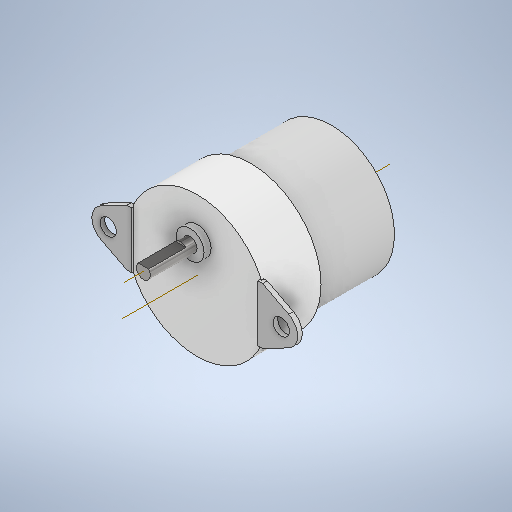
# Autodesk Inventor part: SPG27
Saved by Autodesk Inventor 2025.3 (Build 293356030, 356C)
## iProperties
Created: 2025-08-17
Part Number: SPG27
Material: 一般
Document SubType Name: Modeling
Designer: daisuke
Density: 1 g/cm^3
Appearance: 既定
Author: daisuke
Autodesk Inventor part; units mm, degrees
ref_plane "YZ Plane" through (0, 0, 0) normal (1, 0, 0) x (0, 1, 0)
sketch "スケッチ1" plane through (0, 0, 0) normal (0, 0, 1) x (1, 0, 0)
  circle A0 centre (0, 0) radius 15
  dimension "d0" = 30
  constraints: 1 centre point, 1 coincident
  measures "d0" diameter of A0
extrude "押し出し1" add sketch "スケッチ1" against normal blind 11.5
sketch "スケッチ2" plane through (0, 0, 0) normal (0, 0, 1) x (1, 0, 0)
  circle A0 centre (0, 6.5) radius 3
  point P0 (0, 0)
  dimension "d3" = 6
  dimension "d4" = 6.5
  constraints: 1 centre point, 1 vertical alignment
  measures "d3" diameter of A0
  measures "d4" distance of point (0, 0) A0.centre
extrude "押し出し2" add sketch "スケッチ2" along normal blind 1.5
sketch "スケッチ3" plane through (0, 6.5, 1.5) normal (0, 0, 1) x (1, 0, 0)
  circle A0 centre (0, 0) radius 3 projected
  circle A1 centre (0, 0) radius 1.5
  point P0 (0, -6.5)
  dimension "d7" = 3
  constraints: 1 centre point, 1 coincident
  measures "d7" diameter of A1
extrude "押し出し3" add sketch "スケッチ3" along normal blind 10 contours A1
sketch "スケッチ4" plane through (0, 0, -11.5) normal (0, 0, -1) x (-1, 0, 0)
  circle A0 centre (0, 0) radius 13.5
  dimension "d10" = 27
  constraints: 1 centre point, 1 coincident
  measures "d10" diameter of A0
extrude "押し出し4" add sketch "スケッチ4" along normal blind 17.2
sketch "スケッチ6" plane through (0, 6.5, 11.5) normal (0, 0, 1) x (1, 0, 0)
  circle A0 centre (0, 0) radius 1.5 projected
  line L0 (-1.118, 1) -> (1.118, 1)
  point P0 (0, -6.5)
  dimension "d21" = 1
  constraints: 2 end point, 2 point on circle, 1 horizontal
  measures "d21" distance from line of L0 A0.centre
extrude "押し出し6" cut sketch "スケッチ6" against normal blind 8 contours L0 A0 picked at (-0.0599, 1.1631)
ref_plane "作業平面1" through (0, 0, 0.5) normal (0, 0, 1) x (1, 0, 0)
sketch "スケッチ7" plane through (0, 0, 0.5) normal (0, 0, 1) x (1, 0, 0)
  line L0 (0, 21.4774) -> (0, -21.4774) construction
  line L1 (-14.5, 6) -> (-13.5, 6)
  line L2 (-13.5, 6) -> (-13.5, -6)
  line L3 (-13.5, -6) -> (-14.5, -6)
  line L4 (-14.5, -6) -> (-14.5, 6)
  line L5 (13.5, 6) -> (14.5, 6)
  line L6 (14.5, 6) -> (14.5, -6)
  line L7 (14.5, -6) -> (13.5, -6)
  line L8 (13.5, -6) -> (13.5, 6)
  circle A0 centre (-18.5, 0) radius 1.75
  circle A1 centre (18.5, 0) radius 1.75
  circle A2 centre (-18.5, 0) radius 3.5
  circle A3 centre (18.5, 0) radius 3.5
  line L9 (-14.5, 6) -> (-20.1038, 3.1109)
  line L10 (-20.1038, -3.1109) -> (-14.5, -6)
  line L11 (14.5, 6) -> (20.1038, 3.1109)
  line L12 (20.1038, -3.1109) -> (14.5, -6)
  point P0 (0, 0)
  point P1 (0, 0)
  point P2 (-13.5, 0)
  point P3 (13.5, 0)
  dimension "d25" = 1
  dimension "d26" = 12
  dimension "d27" = 29
  dimension "d28" = 3.5
  dimension "d29" = 37
  dimension "d30" = 7
  constraints: 26 end point, 4 centre point, 4 horizontal alignment, 4 parallel, 4 point on circle, 4 tangent, 3 coincident, 3 midpoint, 2 equal length, 2 equal radius, 2 horizontal, 2 perpendicular, 1 symmetric about line, 1 vertical, 1 other
  measures "d25" distance of L2.end L3.end
  measures "d26" distance of L1.end L2.end
  measures "d27" distance between parallel lines of L6 L4
  measures "d28" diameter of A0
  measures "d29" distance of A1.centre A0.centre
  measures "d30" diameter of A2
extrude "押し出し7" add sketch "スケッチ7" against normal blind 1
ref_plane "作業平面3" through (-10.25, -17.7535, -28.7) normal (-0.5, -0.866, 0) x (0, 0, -1)
ref_plane "作業平面2" through (0, 0, -28.7) normal (-0.5, -0.866, 0) x (0, 0, -1)
sketch "スケッチ9" plane through (-10.25, -17.7535, -28.7) normal (-0.5, -0.866, 0) x (0, 0, -1)
  line L0 (-11.8, -5.25) -> (-8.1, -5.25)
  line L1 (-8.1, -5.25) -> (-8.1, 5.25)
  line L2 (-8.1, 5.25) -> (-11.8, 5.25)
  line L3 (-11.8, 5.25) -> (-11.8, -5.25)
  line L4 (-29.2, -15.855) -> (-29.2, -9.5574) projected
  point P0 (-28.7, 0)
  point P1 (-11.8, 0)
  dimension "d35" = 3.7
  dimension "d36" = 10.5
  dimension "d37" = 17.4
  constraints: 8 end point, 2 parallel, 1 horizontal, 1 horizontal alignment, 1 midpoint, 1 perpendicular
  measures "d35" distance of L2.end L1.end
  measures "d36" distance of L1.end L0.end
  measures "d37" distance between parallel lines of L3 L4
extrude "押し出し8" add sketch "スケッチ9" against normal blind 4
sketch "スケッチ10" plane through (-8.25, -14.2894, -28.7) normal (0.5, 0.866, 0) x (0.866, -0.5, 0)
  line L0 (-6, -4.9) -> (6, -4.9)
  line L1 (6, -4.9) -> (6, -14.3)
  line L2 (6, -14.3) -> (-6, -14.3)
  line L3 (-6, -14.3) -> (-6, -4.9)
  line L4 (-15.855, -29.2) -> (-9.5574, -29.2) projected
  point P0 (0, -28.7)
  point P1 (0, -14.3)
  dimension "d40" = 12
  dimension "d41" = 9.4
  dimension "d42" = 14.9
  constraints: 8 end point, 2 parallel, 1 horizontal, 1 midpoint, 1 perpendicular, 1 vertical alignment
  measures "d40" distance of L1.end L2.end
  measures "d41" distance of L0.end L1.end
  measures "d42" distance between parallel lines of L2 L4
extrude "押し出し9" add sketch "スケッチ10" along normal blind 4
